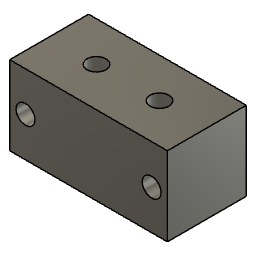
LaserSaftyInterlockDoorBelt v1 (Autodesk Fusion 360 design; units mm, degrees)
Autodesk Fusion 360 part; units mm, degrees
sketch "Sketch1" plane through (0, 0, 0) normal (1, 0, 0) x (0, 0, -1)
  line L0 (12.5, 12.5) -> (-12.5, 12.5)
  line L1 (-12.5, 12.5) -> (-12.5, -12.5)
  line L2 (-12.5, -12.5) -> (12.5, -12.5)
  line L3 (12.5, -12.5) -> (12.5, 12.5)
  line L4 (12.5, 12.5) -> (-12.5, -12.5) construction
  line L5 (-12.5, 12.5) -> (12.5, -12.5) construction
  dimension "d1" = 25
  dimension "d2" = 25
  constraint horizontal L0
  constraint perpendicular L0 L1
  constraint parallel L0 L2
  constraint parallel L1 L3
  constraint coincident L4 origin
  constraint coincident L5 origin
extrude "Extrude1" add sketch "Sketch1" along normal blind 50
sketch "Sketch2" plane through (0, 0, 12.5) normal (0, 0, 1) x (1, 0, 0)
  line L0 (0, 12.5) -> (0, -12.5)
  line L1 (0, -12.5) -> (50, -12.5)
  line L2 (50, -12.5) -> (50, 12.5)
  line L3 (50, 12.5) -> (0, 12.5)
  circle A0 centre (5, 0) radius 3
  line L4 (25, 12.5) -> (25, -12.5) construction
  circle A1 centre (45, 0) radius 3
  dimension "d5" = 6
  dimension "d8" = 20
  constraint midpoint L3 L4.start
  constraint midpoint L1 L4.end
  constraint symmetric A0 L4 A1
  measures "d5" diameter of A0
  measures "d8" distance of A0.centre L4
sketch "Sketch3" plane through (0, 12.5, 0) normal (0, 1, 0) x (-1, 0, 0)
  line L0 (0, -12.5) -> (0, 12.5)
  line L1 (0, 12.5) -> (-50, 12.5)
  line L2 (-50, 12.5) -> (-50, -12.5)
  line L3 (-50, -12.5) -> (0, -12.5)
  line L4 (-25, -12.5) -> (-25, 12.5) construction
  circle A0 centre (-15, 0) radius 3
  circle A1 centre (-35, 0) radius 3
  dimension "d9" = 6
  dimension "d10" = 10
  constraint midpoint L3 L4.start
  constraint midpoint L1 L4.end
  constraint symmetric L4 A0 A1
  measures "d9" diameter of A0
  measures "d10" distance of L4 A0.centre
extrude "Extrude2" cut sketch "Sketch3" against normal through all contours A0 | A1
extrude "Extrude3" cut sketch "Sketch2" against normal through all contours A0 | A1
